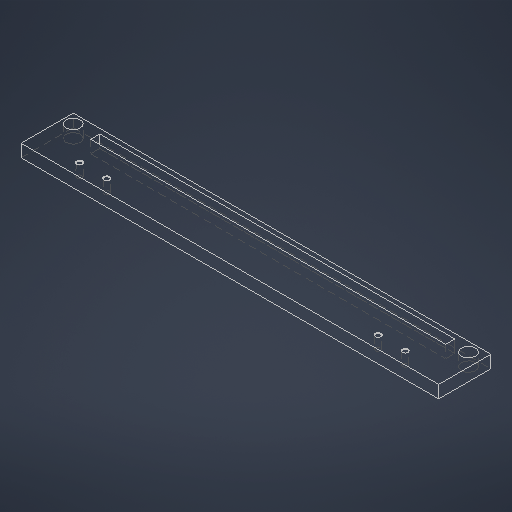
# Autodesk Inventor part: szyna
Saved by Autodesk Inventor 2026.1 (Build 301233020, 233B)
## iProperties
Created: 2026-03-26
Part Number: szyna
Material: Generic
Document SubType Name: Modeling
Designer: Jan
Density: 1 g/cm^3
Appearance: Default
Author: Jan
Autodesk Inventor part; units mm, degrees
ref_plane "YZ Plane" through (0, 0, 0) normal (1, 0, 0) x (0, 1, 0)
ref_plane "XZ Plane" through (0, 0, 0) normal (0, 1, 0) x (-1, 0, 0)
ref_plane "XY Plane" through (0, 0, 0) normal (0, 0, 1) x (1, 0, 0)
sketch "Sketch4" plane through (0, 0, 0) normal (1, 0, 0) x (0, 1, 0)
  line L0 (0, 0) -> (3, 0)
  line L1 (3, 0) -> (3, -4.5)
  line L2 (3, -4.5) -> (0, -4.5)
  line L3 (0, -4.5) -> (0, 0)
  dimension "d21" = 3
  dimension "d22" = 4.5
  constraints: 8 end point, 2 parallel, 1 horizontal, 1 perpendicular
  measures "d21" distance of L1.end L2.end
  measures "d22" distance of L0.end L1.end
extrude "Extrusion2" add sketch "Sketch4" along normal blind 100
sketch "Sketch5" plane through (0, 3, 0) normal (0, 1, 0) x (1, 0, 0)
  circle A0 centre (2.25, 2.25) radius 1.5
  circle A1 centre (96.8723, 2.25) radius 1.5
  line L0 (0, 4.5) -> (0, 0) construction
  line L1 (0, 0) -> (100, 0) construction
  dimension "d25" = 3
  dimension "d26" = 3
  dimension "d27" = 2.25
  dimension "d28" = 2.25
  dimension "d29" = 4.5
  constraints: 2 centre point, 1 horizontal alignment
  measures "d25" diameter of A0
  measures "d26" diameter of A1
  measures "d27" distance from line of L0 A0.centre
  measures "d28" distance from line of L1 A0.centre
  measures "d29" distance of L0.start L0.end
hole "Hole2" at (2.25, 3, -2.25) at (96.8723, 3, -2.25) direction (0, -1, 0) diameter 3.4 depth 8.8 tip angle 118 clearance for "Socket Head Cap Screw ISO 4762" size "M3" standard "ISO"
sketch "Sketch6" plane through (0, 3, 0) normal (0, 1, 0) x (1, 0, 0)
  line L0 (7.5, 1.15) -> (92.5, 1.15)
  line L1 (92.5, 1.15) -> (92.5, 3.35)
  line L2 (92.5, 3.35) -> (7.5, 3.35)
  line L3 (7.5, 3.35) -> (7.5, 1.15)
  line L4 (0, 4.5) -> (100, 4.5) projected
  line L5 (0, 0) -> (100, 0) projected
  line L6 (0, 4.5) -> (0, 0) projected
  dimension "d37" = 85
  dimension "d38" = 2.2
  dimension "d39" = 4.5
  dimension "d40" = 1.15
  dimension "d41" = 7.5
  constraints: 8 end point, 2 parallel, 1 horizontal, 1 perpendicular
  measures "d37" distance of L2.end L1.end
  measures "d38" distance of L1.end L0.end
  measures "d39" distance between parallel lines of L4 L5
  measures "d40" distance from line of L5 L0.start
  measures "d41" distance between parallel lines of L6 L3
extrude "Extrusion3" cut sketch "Sketch6" against normal blind 100
sketch "Sketch7" plane through (0, 0, 0) normal (0, 0, 1) x (1, 0, 0)
  line L0 (0, 0) -> (100, 0)
  line L1 (100, 0) -> (100, 3)
  line L2 (100, 3) -> (0, 3)
  line L3 (0, 3) -> (0, 0)
  constraints: 8 end point, 2 parallel, 1 horizontal, 1 perpendicular
extrude "Extrusion4" add sketch "Sketch7" along normal blind 8
sketch "Sketch8" plane through (0, 3, -4.5) normal (0, 1, 0) x (1, 0, 0)
  line L0 (11, -9.5) -> (89, -9.5) construction
  line L1 (0, 0) -> (0, -12.5) projected
  line L2 (-1, -16) -> (89, -16) construction
  line L3 (-1, -17) -> (89, -17) construction
  line L4 (89, -15) -> (-1, -15) construction
  arc A0 (-1, -15) -> (-1, -17) centre (-1, -16) ccw construction
  arc A1 (89, -17) -> (89, -15) centre (89, -16) ccw construction
  circle A2 centre (11, -9.5) radius 1
  circle A3 centre (89, -9.5) radius 1
  circle A4 centre (82.5, -9.5) radius 1
  circle A5 centre (17.5, -9.5) radius 1
  point P0 (0, -4.5)
  point P1 (50, -9.5)
  point P2 (44, -16)
  dimension "d47" = 78
  dimension "d48" = 50
  dimension "d49" = 2
  dimension "d50" = 90
  dimension "d51" = 6.5
  dimension "d54" = 9.5
  dimension "d55" = 2
  dimension "d56" = 2
  dimension "d57" = 2
  dimension "d58" = 2
  dimension "d59" = 6.5
  dimension "d60" = 6.5
  constraints: 12 end point, 6 centre point, 4 point on circle, 4 tangent, 2 coincident, 2 horizontal, 2 midpoint, 2 point on line, 1 parallel, 1 vertical alignment
  measures "d47" distance of L0.start L0.end
  measures "d48" distance from line of L1 point (50, -9.5)
  measures "d49" diameter of A1
  measures "d50" distance of L2.start L2.end
  measures "d51" distance between parallel lines of L0 L2
  measures "d54" vertical distance of L1.start L0.start
  measures "d55" diameter of A2
  measures "d56" diameter of A3
  measures "d57" diameter of A4
  measures "d58" diameter of A5
  measures "d59" distance of A5.centre L0.start
  measures "d60" distance of A3.centre A4.centre
sketch "Sketch9" plane through (0, 0, -4.5) normal (0, -1, 0) x (1, 0, 0)
  point P0 (0, 4.5)
sketch "Sketch10" plane through (0, 0, -4.5) normal (0, -1, 0) x (1, 0, 0)
  point P0 (0, 4.5)
hole "Hole3" at (11, 3, 5) at (17.5, 3, 5) at (82.5, 3, 5) at (89, 3, 5) direction (0, -1, 0) diameter 1.221 depth 5.3 tip angle 118 thread size "M1.6x0.35" class "6H" standard "ISO Metric profile"
chamfer "Chamfer1" distance 0.1 angle 45 4 edges at (11, 3, 4.3895) (17.5, 3, 4.3895) (82.5, 3, 4.3895) (89, 3, 4.3895)
equation "\"d27\" = d28"
equation "\"d28\" = 0.5 * d29"
body "Solid2"
